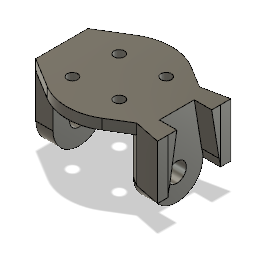
BASE_BRUSHLESS v1 (Autodesk Fusion 360 design; units mm, degrees)
Autodesk Fusion 360 part; units mm, degrees
sketch "Sketch1" plane through (0, 0, 0) normal (0, 1, 0) x (1, 0, 0)
  line L0 (0, 0) -> (23, 0)
  line L1 (0, 0) -> (0, 21)
  line L2 (23, 0) -> (23, 21)
  line L3 (0, 21) -> (-5, 21)
  line L4 (23, 21) -> (28, 21)
  line L5 (28, 21) -> (28, 0)
  line L6 (28, 0) -> (23, 0)
  line L7 (-5, 21) -> (-5, 0)
  line L8 (-5, 0) -> (0, 0)
  line L9 (-5, 0) -> (-5, 15)
  line L10 (-5, 15) -> (28, 15)
  dimension "d1" = 23
  dimension "d2" = 21
  dimension "d3" = 21
  dimension "d4" = 5
  dimension "d5" = 5
  dimension "d6" = 15
  constraint coincident L0.start L1.start
  constraint horizontal L0
  constraint perpendicular L0 L1
  constraint perpendicular L0 L2
  constraint perpendicular L1 L3
  constraint perpendicular L2 L4
  constraint perpendicular L4 L5
  constraint perpendicular L2 L6
  constraint perpendicular L3 L7
  constraint perpendicular L1 L8
  constraint coincident L7 L9.end
  constraint coincident L5 L10.end
  constraint perpendicular L5 L10
  measures "d1" distance of L0.start L0.end
  measures "d2" distance of L0.start L1.end
  measures "d3" distance of L0.end L2.end
  measures "d4" distance of L1.end L3.end
  measures "d5" distance of L2.end L4.end
  measures "d6" distance of L0 L10
extrude "Extrude1" add sketch "Sketch1" along normal blind 6 contours L1 L7 L8 L9 L10 | L2 L5 L6 L10 makes body 1 at (23, 2, -5) makes body 2 at (-5, 2, -10)
extrude "Extrude2" add 2 faces at (24.6667, 6, -10) (-1.6667, 6, -5) along direction (0, 1, 0) blind 20 on bodies 1 2 bodies 1 2
sketch "Sketch2" plane through (28, 0, 0) normal (1, 0, 0) x (0, 0, -1)
  line L0 (0, 0) -> (15, 0)
  line L1 (15, 0) -> (15, 26)
  line L2 (15, 26) -> (0, 26)
  line L3 (0, 26) -> (0, 0)
  line L4 (15, 0) -> (15, 15)
  line L5 (0, 15) -> (15, 15)
  circle A0 centre (7.5, 7.5) radius 2.75
  circle A1 centre (7.5, 7.5) radius 7.5
  line L6 (15, 20) -> (0, 20)
  dimension "d11" = 5.5
  dimension "d12" = 7.5
  dimension "d13" = 7.5
  dimension "d14" = 15
  dimension "d15" = 5
  constraint coincident L0.end L1.start
  constraint coincident L1 L4.end
  constraint perpendicular L0 L4
  constraint coincident L3 L5.start
  constraint perpendicular L1 L5
  constraint concentric A0 A1
  constraint tangent L4 A1
  constraint coincident L1 L6.start
  constraint coincident L3 L6.end
  constraint perpendicular L3 L6
  measures "d11" diameter of A0
  measures "d12" distance of L4 A0.centre
  measures "d13" distance of L0 A0.centre
  measures "d14" distance of L0 L5
  measures "d15" distance of L5 L6
extrude "Extrude3" cut sketch "Sketch2" against normal blind 50 contours L0 L3 A1 | L0 L1 L4 A1 | L1 L2 L3 L6 | A0 bodies 1 2
sketch "Sketch3" plane through (0, 20, 0) normal (0, 1, 0) x (-1, 0, 0)
  line L0 (0, 0) -> (0, -15)
  line L1 (0, -15) -> (5, -15)
  line L2 (5, -15) -> (5, 0)
  line L3 (5, 0) -> (0, 0)
  circle A0 centre (-11.5, -7.5) radius 15
  circle A1 centre (-11.5, -7.5) radius 9.5
  line L4 (5, -15) -> (-28, -15)
  line L5 (-28, -15) -> (-28, 0)
  line L6 (-28, 0) -> (5, 0)
  line L7 (5, 0) -> (5, -15)
  circle A2 centre (-11.5, -7.5) radius 8
  line L8 (-11.5, -7.5) -> (-24, -7.5)
  line L9 (-24, -7.5) -> (-11.5, -7.5)
  line L10 (-11.5, -7.5) -> (-22.1066, -18.1066)
  line L11 (-11.5, -7.5) -> (-0.8934, -18.1066)
  circle A3 centre (-18.2175, -14.2175) radius 1.5
  circle A4 centre (-4.7825, -0.7825) radius 1.5
  circle A5 centre (-5.8431, -13.1569) radius 1.5
  circle A6 centre (-17.1569, -1.8431) radius 1.5
  line L12 (5, -15) -> (-3.6827, -20.3019)
  line L13 (-28, -15) -> (-19.3173, -20.3019)
  line L14 (5, 0) -> (-3.6827, 5.3019)
  line L15 (-28, 0) -> (-19.3173, 5.3019)
  dimension "d18" = 30
  dimension "d19" = 19
  dimension "d20" = 16
  dimension "d21" = 45
  dimension "d22" = 90
  dimension "d23" = 3
  dimension "d25" = 360
  dimension "d26" = 3
  dimension "d28" = 360
  constraint concentric A0 A1
  constraint horizontal L4
  constraint vertical L5
  constraint horizontal L6
  constraint vertical L7
  constraint coincident L1.end L2.start
  constraint concentric A1 A2
  constraint coincident A0.centre A1.centre
  constraint perpendicular L5 L8
  constraint perpendicular L5 L9
  constraint coincident A0 L10.end
  constraint coincident A0 L11.end
  constraint coincident A1 A3.centre
  constraint coincident L10 A3.centre
  constraint coincident A2 A5.centre
  constraint coincident L11 A5.centre
  constraint coincident A0 L12.end
  constraint tangent A0 L12
  constraint coincident A0 L13.end
  constraint tangent A0 L13
  constraint coincident L2.end L3.start
  constraint coincident A0 L14.end
  constraint tangent A0 L14
  constraint parallel L13 L14
  constraint coincident A0 L15.end
  constraint tangent A0 L15
  constraint parallel L12 L15
  measures "d18" diameter of A0
  measures "d19" diameter of A1
  measures "d20" diameter of A2
  measures "d21" angle of L8 L10
  measures "d22" angle of L10 L11
  measures "d23" diameter of A3
  measures "d26" diameter of A5
extrude "Extrude4" add sketch "Sketch3" along normal blind 3 contours L0 L1 L3 A0 L4 L6 | L3 A0 A1 L6 A4 | L0 A1 L4 L6 L11 A4 | L1 A0 L4 L11 | L3 A0 L6 L14 | L1 L2 L3 A0 L4 L6 L7 | L1 A0 L4 L12 | A0 A1 L4 L10 L11 A3 | A1 L4 L11 | A1 L6 A2 A4 | A1 L4 A2 A5 | A1 L4 A2 A3 | A1 A2 A4 A5 | A0 L6 L15 | L6 A2 A4 | A1 L6 A2 A6 | A0 A1 L4 L6 A3 | L4 A2 | L4 A2 L10 L11 A5 | A0 L4 L5 L6 | L6 A2 L8 L9 L11 A5 A6 | L6 A2 | A1 A2 L8 L9 A6 | A0 L4 L13 | A0 L4 L10 A3 | L4 A2 A3 | A1 A2 L8 L9 A3 | A2 L8 L9 L10 bodies 1 2
sketch "Sketch4" plane through (28, 0, 0) normal (1, 0, 0) x (0, 0, -1)
  line L0 (0, 20) -> (0, 7.5)
  arc A0 (0, 7.5) -> (15, 7.5) centre (7.5, 7.5) ccw
  line L1 (15, 7.5) -> (15, 20)
  line L2 (15, 20) -> (15, 23)
  line L3 (15, 23) -> (0, 23)
  line L4 (0, 23) -> (0, 20)
  circle A1 centre (7.5, 7.5) radius 2.75
  circle A2 centre (7.5, 7.5) radius 7.5
  line L5 (7.5, 7.5) -> (7.5, 23)
  line L6 (7.5, 23) -> (12.5, 23)
  line L7 (7.5, 23) -> (2.5, 23)
  line L8 (2.5, 23) -> (0, 7.5)
  line L9 (12.5, 23) -> (15, 7.5)
  dimension "d31" = 15
  dimension "d32" = 5
  dimension "d33" = 5
  constraint concentric A0 A2
  constraint coincident A0.centre A1.centre
  constraint midpoint L3 L5.end
  constraint perpendicular L5 L6
  constraint perpendicular L5 L7
  constraint coincident L0.end A0.start
  constraint coincident A0.end L1.start
  measures "d31" diameter of A2
  measures "d32" distance of L5.end L6.end
  measures "d33" distance of L5.end L7.end
extrude "Extrude5" add sketch "Sketch4" along normal blind 5 contours L0 L3 L4 A2 L8 | L1 L2 L3 A2 L9 bodies 1
sketch "Sketch5" plane through (0, 23, 0) normal (0, 1, 0) x (-1, 0, 0)
  circle A0 centre (-18.2175, -14.2175) radius 1.5
  circle A1 centre (-5.8431, -13.1569) radius 1.5
  circle A2 centre (-17.1569, -1.8431) radius 1.5
  circle A3 centre (-4.7825, -0.7825) radius 1.5
  line L0 (-28, -15) -> (-19.3173, -20.3019)
  arc A4 (-19.3173, -20.3019) -> (-3.6827, -20.3019) centre (-11.5, -7.5) ccw
  line L1 (-3.6827, -20.3019) -> (5, -15)
  line L2 (5, -15) -> (5, 0)
  line L3 (5, 0) -> (-3.6827, 5.3019)
  arc A5 (-3.6827, 5.3019) -> (-19.3173, 5.3019) centre (-11.5, -7.5) ccw
  line L4 (-19.3173, 5.3019) -> (-28, 0)
  line L5 (-28, 0) -> (-33, 0)
  line L6 (-33, 0) -> (-33, -2.5)
  line L7 (-33, -2.5) -> (-28, -2.5)
  line L8 (-28, -2.5) -> (-28, -12.5)
  line L9 (-28, -12.5) -> (-33, -12.5)
  line L10 (-33, -12.5) -> (-33, -15)
  line L11 (-33, -15) -> (-28, -15)
  line L12 (-23, -15) -> (-28, -15)
  line L13 (-25.5, -15) -> (-25.5, -18.0532)
  line L14 (-25.5, -18.0532) -> (-33, -18.0532)
  line L15 (-33, -18.0532) -> (-33, -15)
  line L16 (-23, 0) -> (-28, 0)
  line L17 (-25.5, 0) -> (-25.5, 3.0532)
  line L18 (-25.5, 3.0532) -> (-33, 3.0532)
  line L19 (-33, 3.0532) -> (-33, 0)
  line L20 (-28, 0) -> (-25.5, 1.5266)
  line L21 (-28, -15) -> (-25.5, -16.5266)
  line L22 (-25.5, -16.5266) -> (-33, -18.0532)
  line L23 (-33, 3.0532) -> (-25.5, 1.5266)
  constraint coincident L0.start L11.end
  constraint parallel L11 L12
  constraint midpoint L12 L13.start
  constraint perpendicular L12 L13
  constraint perpendicular L13 L14
  constraint coincident L10.end L11.start
  constraint coincident L4.end L5.start
  constraint perpendicular L13 L16
  constraint midpoint L16 L17.start
  constraint perpendicular L16 L17
  constraint perpendicular L17 L18
  constraint coincident L5.end L6.start
  constraint midpoint L17 L20.end
  constraint midpoint L13 L21.end
extrude "Extrude6" add sketch "Sketch5" against normal blind 15.5 contours L0 L11 L15 L21 L22 | L4 L5 L19 L20 L23 bodies 1
sketch "Sketch6" plane through (0, 20, 0) normal (0, -1, 0) x (1, 0, 0)
  circle A0 centre (4.7825, -0.7825) radius 1.5
  circle A1 centre (17.1569, -1.8431) radius 1.5
  circle A2 centre (5.8431, -13.1569) radius 1.5
  circle A3 centre (18.2175, -14.2175) radius 1.5
  line L0 (-5, 0) -> (0, 0)
  line L1 (0, 0) -> (0, -15)
  line L2 (0, -15) -> (-5, -15)
  line L3 (-5, -15) -> (3.6827, -20.3019)
  arc A4 (3.6827, -20.3019) -> (19.3173, -20.3019) centre (11.5, -7.5) ccw
  line L4 (19.3173, -20.3019) -> (25.5, -16.5266)
  line L5 (25.5, -16.5266) -> (28, -15)
  line L6 (28, -15) -> (23, -15)
  line L7 (23, -15) -> (23, 0)
  line L8 (23, 0) -> (28, 0)
  line L9 (28, 0) -> (25.5, 1.5266)
  line L10 (25.5, 1.5266) -> (19.3173, 5.3019)
  arc A5 (19.3173, 5.3019) -> (3.6827, 5.3019) centre (11.5, -7.5) ccw
  line L11 (3.6827, 5.3019) -> (-5, 0)
  line L12 (25.5, 1.5266) -> (25.5, 0)
  line L13 (25.5, -16.5266) -> (25.5, -15)
  line L14 (28, -15) -> (25.5, -15)
  line L15 (25.5, -16.5266) -> (28, -15)
  line L16 (25.5, 1.5266) -> (28, 0)
  line L17 (28, 0) -> (25.5, 0)
  constraint coincident L9.end L10.start
  constraint midpoint L8 L12.end
  constraint coincident L4.end L5.start
  constraint midpoint L6 L13.end
  constraint coincident L5.end L6.start
  constraint coincident L8.end L9.start
extrude "Extrude7" add sketch "Sketch6" along normal blind 15.5 contours L8 L9 L12 L16 L17 | L5 L6 L13 L14 L15 bodies 1
extrude "Extrude8" cut 2 faces at (26.3333, 4.5, -15.5089) (26.3333, 4.5, 0.5089) along direction (0, 1, 0) blind 3 on bodies 1 bodies 1
sketch "Sketch7" plane through (0, 20, 0) normal (0, -1, 0) x (1, 0, 0)
  line L0 (25.5, -16.5266) -> (25.5, -15)
  line L1 (25.5, -15) -> (23, -15)
  line L2 (23, -15) -> (23, 0)
  line L3 (23, 0) -> (25.5, 0)
  line L4 (25.5, 0) -> (25.5, 1.5266)
  line L5 (25.5, 1.5266) -> (19.3173, 5.3019)
  arc A0 (19.3173, 5.3019) -> (3.6827, 5.3019) centre (11.5, -7.5) ccw
  line L6 (3.6827, 5.3019) -> (-5, 0)
  line L7 (-5, 0) -> (0, 0)
  line L8 (0, 0) -> (0, -15)
  line L9 (0, -15) -> (-5, -15)
  line L10 (-5, -15) -> (3.6827, -20.3019)
  arc A1 (3.6827, -20.3019) -> (19.3173, -20.3019) centre (11.5, -7.5) ccw
  line L11 (19.3173, -20.3019) -> (25.5, -16.5266)
  circle A2 centre (18.2175, -14.2175) radius 1.5
  circle A3 centre (5.8431, -13.1569) radius 1.5
  circle A4 centre (17.1569, -1.8431) radius 1.5
  circle A5 centre (4.7825, -0.7825) radius 1.5
  line L12 (25.5, -16.5266) -> (23, -15)
  line L13 (25.5, -15) -> (25.5, -16.5266)
  line L14 (25.5, -15) -> (23, -15)
  line L15 (23, 0) -> (25.5, 1.5266)
  line L16 (25.5, 1.5266) -> (25.5, 0)
  line L17 (25.5, 0) -> (23, 0)
  constraint coincident L0.start L11.end
  constraint coincident L1.end L2.start
  constraint coincident L0.end L1.start
  constraint coincident L2.end L3.start
  constraint coincident L4.end L5.start
  constraint coincident L3.end L4.start
extrude "Extrude9" add sketch "Sketch7" along normal blind 12.5 contours L0 L1 L12 L13 L14 | L3 L4 L15 L16 L17 bodies 1
